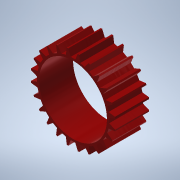
# Autodesk Inventor part: NASA-20-TRD-01
Saved by Autodesk Inventor 2020 (Build 240168000, 168)
## iProperties
Created: 2019-09-21
Part Number: NASA-20-TRD-01
Material: PET Plastic
Document SubType Name: Modeling
Designer: Rick Szalay
Density: 1.541 g/cm^3
Appearance: Red
Author: Rick Szalay
Autodesk Inventor part; units mm, degrees
ref_plane "YZ Plane" through (0, 0, 0) normal (1, 0, 0) x (0, 1, 0)
ref_plane "XZ Plane" through (0, 0, 0) normal (0, 1, 0) x (-1, 0, 0)
ref_plane "XY Plane" through (0, 0, 0) normal (0, 0, 1) x (1, 0, 0)
sketch "Sketch1" plane through (0, 0, 0) normal (0, 0, 1) x (1, 0, 0)
  circle A0 centre (0, 0) radius 101.6
  circle A1 centre (0, 0) radius 127
  dimension "d0" = 203.2
  dimension "d1" = 25.4
  constraints: 2 centre point, 1 coincident
  measures "d0" diameter of A0
  measures "d1" radial gap between concentric circles of A0 A1
extrude "Extrusion1" add sketch "Sketch1" along normal mid plane 101.6
sketch "Sketch2" plane through (0, 0, 50.8) normal (0, 0, 1) x (1, 0, 0)
  circle A0 centre (0, 0) radius 127 projected
  line L0 (-14.3768, 126.1836) -> (-6.8242, 107.95)
  line L1 (-6.8242, 107.95) -> (6.8242, 107.95)
  line L2 (6.8242, 107.95) -> (14.3768, 126.1836)
  line L3 (0, 107.95) -> (0, 128.4311) construction
  line L4 (-14.3768, 126.1836) -> (0, 0) construction
  line L5 (0, 0) -> (14.3768, 126.1836) construction
  arc A1 (14.3768, 126.1836) -> (-14.3768, 126.1836) centre (0, 0) ccw
  dimension "d4" = 19.05
  dimension "d5" = 45
  dimension "d6" = 13
  constraints: 12 end point, 4 point on circle, 1 centre point, 1 concentric, 1 horizontal, 1 midpoint, 1 vertical, 1 vertical alignment, 1 other
  measures "d4" distance edge to line of A0 L1
  measures "d5" angle of L0 L2
  measures "d6" angle of L4 L5
extrude "Extrusion2" cut sketch "Sketch2" against normal through all contours L2 L1 L0 A0 picked at (1.6005, 114.2697)
pattern_circular "Circular Pattern1" count 24 over 360 about axis through (0, 0, 0) along (0, 0, 1) of "Extrusion2"
body "Solid1"
